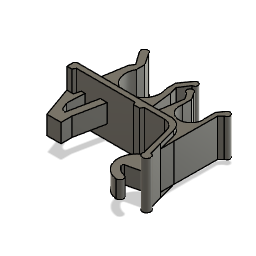
Trooper_Hood_Prop_Holder (Autodesk Fusion 360 design; units mm, degrees)
Autodesk Fusion 360 part; units mm, degrees
note: some values were not read from the file. Set by a fixed rule: which sketch regions a step uses.
sketch "Sketch1" plane through (0, 0, 0) normal (0, 1, 0) x (1, 0, 0)
  circle A0 centre (0, 0) radius 5.5245
  circle A1 centre (-8.3413, 8.723) radius 1.1194
  circle A2 centre (8.2886, 8.0328) radius 0.9582
  circle A3 centre (9.6564, 5.164) radius 1.0287
  line L0 (5.0806, 2.1697) -> (5.0806, 5.1735)
  line L1 (5.0806, 5.1735) -> (7.5076, 8.588)
  line L2 (8.3228, 7.0753) -> (6.3824, 4.0232)
  line L3 (6.3824, 4.0232) -> (7.0069, 1.6241)
  line L4 (7.0069, 1.6241) -> (8.0257, -6.3622)
  line L5 (8.0257, -6.3622) -> (9.5046, -6.3622)
  line L6 (9.5046, -6.3622) -> (10.7841, 1.9482)
  line L7 (10.7841, 1.9482) -> (10.8788, 2.2561)
  line L8 (10.8788, 2.2561) -> (9.572, 4.1388)
  circle A4 centre (15.6792, -0.5867) radius 3.7465
  line L9 (10.6759, 5.3009) -> (12.0353, 3.2345)
  line L10 (12.0353, 3.2345) -> (12.0353, 0.2841)
  line L11 (-7.2674, 9.0389) -> (-4.8494, 5.3631)
  line L12 (-4.8494, 5.3631) -> (-4.8494, 2.6464)
  line L13 (-9.2541, 8.0752) -> (-6.3655, 4.0047)
  line L14 (-6.3655, 4.0047) -> (-7.2567, 2.5114)
  line L15 (-7.2567, 2.5114) -> (-8.67, -6.2965)
  line L16 (19.3393, 3.3813) -> (20.7205, 5.4216)
  circle A5 centre (21.5724, 4.8449) radius 1.0287
  line L17 (20.676, -15.1957) -> (20.6321, -10.9388)
  line L18 (20.6321, -10.9388) -> (20.7199, 2.7537)
  line L19 (20.7199, 2.7537) -> (21.7328, 3.8288)
  line L20 (19.3393, 3.3813) -> (19.3581, 0.1219)
  line L21 (-8.67, -6.2965) -> (8.0257, -6.3622)
  line L22 (9.5046, -6.3622) -> (14.58, -6.3622)
  line L23 (20.676, -15.1957) -> (19.162, -9.4944)
  arc A6 (19.162, -9.4944) -> (14.58, -6.3622) centre (15.0549, -10.585) ccw
  line L24 (-8.67, -6.2965) -> (-0.3221, -6.3294)
  line L25 (-15.1739, -7.0327) -> (-15.1739, -8.8646)
  line L26 (-15.1739, -8.8646) -> (-13.6149, -8.8646)
  line L27 (-13.6149, -8.8646) -> (-13.1861, -7.9487)
  line L28 (-13.1861, -7.9487) -> (5.3274, -7.9487)
  line L29 (5.3274, -7.9487) -> (5.8341, -8.8646)
  line L30 (5.8341, -8.8646) -> (7.7439, -8.8646)
  line L31 (7.7439, -8.8646) -> (8.2896, -7.9487)
  line L32 (8.2896, -7.9487) -> (14.6426, -7.9487)
  line L33 (-8.67, -6.2965) -> (-0.3221, -6.3294)
  line L34 (-14.3937, -6.274) -> (-8.67, -6.2965)
  arc A7 (-14.3937, -6.274) -> (-15.1739, -7.0327) centre (-14.4149, -7.0327) ccw
  arc A8 (17.9946, -10.5406) -> (14.6426, -7.9487) centre (14.6426, -11.412) ccw
  circle A9 centre (21.699, -20.6353) radius 1.2801
  line L35 (20.676, -15.1957) -> (21.8628, -19.3658)
  line L36 (17.9946, -10.5406) -> (20.5015, -20.1831)
  arc A10 (19.248, -15.3618) -> (18.6571, -27.2222) centre (19.3333, -21.311) ccw
  arc A11 (18.6571, -27.2222) -> (19.248, -25.0006) centre (18.616, -26.0219) ccw
  arc A12 (15.8119, -22.779) -> (19.248, -25.0006) centre (19.8724, -20.2669) ccw
  arc A13 (16.0915, -22.0573) -> (15.8119, -22.779) centre (16.3252, -22.5629) ccw
  line L37 (16.0915, -22.0573) -> (20.4797, -21.0248)
  line L38 (-5.6013, -7.9487) -> (-7.4672, -17.2088)
  line L39 (-5.273, -17.2088) -> (-3.4071, -7.9487)
  arc A14 (-11.2863, -6.2862) -> (-8.0974, -2.7283) centre (-12.4572, -2.0288) ccw
  arc A15 (7.4405, 1.884) -> (6.3824, 4.0232) centre (3.3656, 1.1998) ccw
  arc A16 (10.4867, 2.8211) -> (9.2772, 0.0735) centre (13.841, -0.2954) ccw
  arc A17 (8.1489, -2.7078) -> (8.9099, -2.6553) centre (8.5286, -2.6693) ccw
  line L40 (7.4405, 1.884) -> (8.1489, -2.7078)
  line L41 (9.2772, 0.0735) -> (8.9099, -2.6553)
  line L42 (-5.273, -17.2088) -> (-5.273, -20.6487)
  line L43 (-5.273, -20.6487) -> (-9.718, -20.6487)
  line L44 (-9.718, -20.6487) -> (-13.2025, -10.8993)
  line L45 (-13.2025, -10.8993) -> (-11.133, -10.8993)
  arc A18 (-8.8014, -16.504) -> (-7.4672, -17.2088) centre (-7.4317, -15.5263) ccw
  line L46 (-11.133, -10.8993) -> (-10.603, -8.9308)
  line L47 (-10.603, -8.9308) -> (-9.3916, -8.9308)
  line L48 (-9.3916, -8.9308) -> (-9.7064, -14.3939)
  line L49 (-8.8014, -16.504) -> (-9.7064, -14.3939)
  dimension "d1" = 11.049
  dimension "d2" = 7.493
  dimension "d3" = 2.0574
  dimension "d4" = 2.9504
  dimension "d6" = 2.4735
  dimension "d7" = 2.4638
  dimension "d8" = 146.662
  dimension "d10" = 2.0574
  dimension "d11" = 128.128
  dimension "d12" = 2.2918
  dimension "d28" = 12.7
  dimension "d29" = 4.445
  dimension "d32" = 9.779
  constraint coincident A0.centre origin
  constraint coincident A0 L0.start
  constraint vertical L0
  constraint coincident A2 L1.end
  constraint tangent A2 L1
  constraint coincident A2 L2.start
  constraint coincident A3 L8.end
  constraint coincident A3 L9.start
  constraint coincident A4 L10.end
  constraint vertical L10
  constraint coincident A1 L11.start
  constraint parallel L9 L11
  constraint coincident A0 L12.end
  constraint parallel L10 L12
  constraint coincident A1 L13.start
  constraint tangent A1 L13
  constraint coincident A5 L19.end
  constraint coincident A4 L20.end
  constraint tangent L23 A6
  constraint parallel L21 L24
  constraint vertical L25
  constraint perpendicular L25 L26
  constraint perpendicular L25 L28
  constraint parallel L28 L30
  constraint parallel L30 L32
  constraint parallel L21 L33
  constraint parallel L21 L34
  constraint tangent L25 A7
  constraint tangent L32 A8
  constraint coincident A9 L35.end
  constraint coincident A9 L36.end
  constraint tangent A8 L36
  constraint midpoint L36 A10.start
  constraint tangent A10 A12
  constraint coincident A9 L37.end
  constraint coincident L28 L38.start
  constraint coincident L28 L39.end
  constraint parallel L38 L39
  constraint tangent L15 A14
  constraint coincident L15 A14.end
  constraint coincident L8 A16.start
  constraint coincident L34 A14.start
  constraint coincident L16.end A5
  constraint tangent L16 A5
  constraint perpendicular L42 L43
  constraint parallel L43 L45
  constraint parallel L45 L47
  measures "d1" diameter of A0
  measures "d2" diameter of A4
  measures "d3" diameter of A3
  measures "d4" distance of L9.end L10.end
  measures "d6" distance of L9.start L9.end
  measures "d7" distance of L16.start L16.end
  measures "d8" angle of L9 L10
  measures "d10" diameter of A5
  measures "d11" angle of L7 L8
  measures "d12" distance of L7.end L8.end
  measures "d28" distance of L28 L42.end
  measures "d29" distance of L42.end L43.end
  measures "d32" distance of L27.end L39.end
extrude "Extrude2" add sketch "Sketch1" along normal mid plane 14.859 contours L5 L21 L22 L23 A6 L24 L25 L26 L27 L28 L29 L30 L31 L32 L33 L34 A7 A8 A9 L35 L36 | A9
extrude "Extrude3" add sketch "Sketch1" along normal mid plane 5.842 contours L28 L38 L39 L42 L43 L44 L45 A18 L46 L47 L48 L49
extrude "Extrude4" add sketch "Sketch1" along normal mid plane 11.811 contours A0 A1 A2 L0 L1 L2 L3 L4 L11 L12 L13 L14 L15 L21 L24 L33 | A2 | A3 L6 L7 L8 A4 L9 L10 L16 A5 L17 L18 L19 L20 L22 L23 A6 | A3 | A5
extrude "Extrude5" add sketch "Sketch1" along normal mid plane 2.032 contours L3 L4 L5 L6 L7 L8 A15 A16 A17 L40 L41 | L15 L34 A14
extrude "Extrude6" add sketch "Sketch1" along normal mid plane 5.461 contours A9 L36 A10 A11 A12 A13 L37
extrude "Extrude7" add sketch "Sketch1" along normal mid plane 11.811 contours A1
named bodies: "Hood_Prop_Clip"
